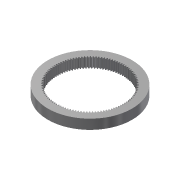
# Autodesk Inventor part: ring2
Saved by Autodesk Inventor 2018 (Build 220112000, 112)
## iProperties
Created: 2019-12-31
Part Number: ring2
Material: Steel
Document SubType Name: Modeling
Designer: louis
Categories: <?xml version="1.0" encoding="UTF-16"?> <MemberInstance><Categories><FamilyTemplate><FamilyTemplateParameter ValueType="xs:double" Id="1" ObjectReferenceKey="da_z" ObjectType="kUserParameterObject"/><FamilyTemplateParameter ValueType="xs:double" Id="2" ObjectReferenceKey="da_b" ObjectType="kUserParameterObject"/><FamilyTemplateParameter ValueType="xs:double" Id="3" ObjectReferenceKey="da_beta" ObjectType="kUserParameterObject"/><FamilyTemplateParameter ValueType="xs:double" Id="4" ObjectReferenceKey="da_da" ObjectType="kUserParameterObject"/><FamilyTemplateParameter ValueType="xs:double" Id="5" ObjectReferenceKey="da_aw" ObjectType="kUserParameterObject"/><FamilyTemplateParameter ValueType="xs:string" Id="6" ObjectReferenceKey="EAIAABAAAACIAQAAAAAAAIAAAAAAAAAA" ObjectType="83910656" SubObjectId="SurfaceGeometry"/></FamilyTemplate><ParamToTemplateMap><ParamToTemplate CategoryParameter="//CategoryParameter[@InternalName='046C89C9-8512-4d59-83FE-43B91F4F132A']" TemplateParameter="1"/><ParamToTemplate CategoryParameter="//CategoryParameter[@InternalName='2552DF32-E462-4b46-AEBF-C6C7768E72AC']" TemplateParameter="2"/><ParamToTemplate CategoryParameter="//CategoryParameter[@InternalName='C9EE641D-15FC-4fae-A226-E94C4372FDD7']" TemplateParameter="3"/><ParamToTemplate><ParamToTemplate CategoryParameter="//CategoryParameter[@InternalName='00B6519A-459B-49c7-AD84-2E56D39A5744']" ConstantValue="0.000000"/></ParamToTemplate><ParamToTemplate><ParamToTemplate CategoryParameter="//CategoryParameter[@InternalName='04B31F0E-C7A6-4894-AA32-9629BEFACF47']" ConstantValue="1.000000"/></ParamToTemplate><ParamToTemplate><ParamToTemplate CategoryParameter="//CategoryParameter[@InternalName='43CBEC2E-7847-49e7-A936-2F7889FCB2D9']" ConstantValue="0.250000"/></ParamToTemplate><ParamToTemplate><ParamToTemplate CategoryParameter="//CategoryParameter[@InternalName='B1EFC894-105D-4ebd-86BF-FA20ED196853']" ConstantValue="0.350000"/></ParamToTemplate><ParamToTemplate><ParamToTemplate CategoryParameter="//CategoryParameter[@InternalName='51175063-3D10-4879-93E8-6246FE8B403D']" ConstantValue="2060000000.000000"/></ParamToTemplate><ParamToTemplate><ParamToTemplate CategoryParameter="//CategoryParameter[@InternalName='A3A52E27-4454-46a9-B0BD-C932399B70AF']" ConstantValue="0.300000"/></ParamToTemplate><ParamToTemplate><ParamToTemplate CategoryParameter="//CategoryParameter[@InternalName='91B76062-C214-41d9-B1B9-14D2AB99603D']" ConstantValue="0.100000"/></ParamToTemplate><ParamToTemplate><ParamToTemplate CategoryParameter="//CategoryParameter[@InternalName='374E806E-8B8A-4dda-A9AA-1039D6500AD2']" ConstantValue="10.000000"/></ParamToTemplate><ParamToTemplate><ParamToTemplate CategoryParameter="//CategoryParameter[@InternalName='2D373A89-B862-43d6-8D0B-0CBF12AB9F6C']" ConstantValue="0.349066"/></ParamToTemplate><ParamToTemplate CategoryParameter="//CategoryParameter[@InternalName='37777632-D6A2-4fac-9D53-DB8ACD95C989']" TemplateParameter="4"/><ParamToTemplate CategoryParameter="//CategoryParameter[@InternalName='FD1017F1-B727-4f7e-9707-0F86F1FF9423']" TemplateParameter="5"/><ParamToTemplate><ParamToTemplate CategoryParameter="//CategoryParameter[@InternalName='9E1B4470-B2D3-4ff1-B813-535BB4CDF51A']" ConstantValue="3520000.000000"/></ParamToTemplate><ParamToTemplate><ParamToTemplate CategoryParameter="//CategoryParameter[@InternalName='F8452263-BFF6-458c-9FB1-07C4B99E95CD']" ConstantValue="11400000.000000"/></ParamToTemplate><ParamToTemplate><ParamToTemplate CategoryParameter="//CategoryParameter[@InternalName='3E3BB259-FD49-497f-8171-6EBC954A3479']" ConstantValue="2.000000"/></ParamToTemplate><ParamToTemplate CategoryParameter="//CategoryParameter[@InternalName='27C3BAF2-7550-4e4b-AE2C-0DB134B7D9B7']" TemplateParameter="6"/></ParamToTemplateMap><Category DisplayName="Gear" InternalName="DC85795E-93AB-48d5-8EEE-5A27447B64BD" Mnemonic="Gear"><CategoryParameter DisplayName="z" InternalName="046C89C9-8512-4d59-83FE-43B91F4F132A" Mnemonic="z"/><CategoryParameter DisplayName="b" InternalName="2552DF32-E462-4b46-AEBF-C6C7768E72AC" Mnemonic="b"/><CategoryParameter DisplayName="||b|" InternalName="C9EE641D-15FC-4fae-A226-E94C4372FDD7" Mnemonic="beta"/><CategoryParameter DisplayName="x" InternalName="00B6519A-459B-49c7-AD84-2E56D39A5744" Mnemonic="x"/><CategoryParameter DisplayName="a*" InternalName="04B31F0E-C7A6-4894-AA32-9629BEFACF47" Mnemonic="a"/><CategoryParameter DisplayName="c*" InternalName="43CBEC2E-7847-49e7-A936-2F7889FCB2D9" Mnemonic="c"/><CategoryParameter DisplayName="r|.f|*" InternalName="B1EFC894-105D-4ebd-86BF-FA20ED196853" Mnemonic="rf"/><CategoryParameter DisplayName="E" InternalName="51175063-3D10-4879-93E8-6246FE8B403D" Mnemonic="E"/><CategoryParameter DisplayName="||m|" InternalName="A3A52E27-4454-46a9-B0BD-C932399B70AF" Mnemonic="mi"/><Category DisplayName="SpurGear" InternalName="26C5A22E-A91E-4dfd-A3B3-23CCAFAE1764" Mnemonic="SpurGear"><CategoryParameter DisplayName="m" InternalName="91B76062-C214-41d9-B1B9-14D2AB99603D" Mnemonic="m"/><CategoryParameter DisplayName="P" InternalName="374E806E-8B8A-4dda-A9AA-1039D6500AD2" Mnemonic="PP"/><CategoryParameter DisplayName="||a|" InternalName="2D373A89-B862-43d6-8D0B-0CBF12AB9F6C" Mnemonic="alpha"/><CategoryParameter DisplayName="d|.a|" InternalName="37777632-D6A2-4fac-9D53-DB8ACD95C989" Mnemonic="da"/><CategoryParameter DisplayName="a|.w|" InternalName="FD1017F1-B727-4f7e-9707-0F86F1FF9423" Mnemonic="aw"/><CategoryParameter DisplayName="||s||.Flim|" InternalName="9E1B4470-B2D3-4ff1-B813-535BB4CDF51A" Mnemonic="sFlim"/><CategoryParameter DisplayName="||s||.Hlim|" InternalName="F8452263-BFF6-458c-9FB1-07C4B99E95CD" Mnemonic="sHlim"/><CategoryParameter DisplayName="類型" InternalName="3E3BB259-FD49-497f-8171-6EBC954A3479" Mnemonic="type"/><CategoryParameter DisplayName="PitchDiameter" InternalName="27C3BAF2-7550-4e4b-AE2C-0DB134B7D9B7" Mnemonic="IDS_PITCHDIAM"/></Category></Category></Categories></MemberInstance>
Density: 1 g/cm^3
Appearance: Steel
CustomPartVersion: 1
Author: louis
Autodesk Inventor part; units mm, degrees
sketch "Sketch1" plane through (0, 0, 0) normal (0, 0, 1) x (1, 0, 0)
  circle A0 centre (0, 0) radius 53.5
  dimension "d0" = 107
  constraints: 1 centre point
  measures "d0" diameter of A0
extrude "Extrusion1" add sketch "Sketch1" along normal blind 15
ref_plane "Work Plane2" through (0, 0, 7.5) normal (0, 0, 1) x (1, 0, 0)
sketch "Sketch2" plane through (0, 0, 0) normal (0, 0, -1) x (-1, 0, 0)
  circle A0 centre (0, 0) radius 53.5 projected
  circle A1 centre (0, 0) radius 52.5
  dimension "d3" = 105
  constraints: 1 centre point, 1 coincident
  measures "d3" diameter of A1
surface extrude "節圓直徑" sketch "Sketch2" against normal through all shown no curves A1
ref_plane "Work Plane8" through (0, 0, 0) normal (0.9995524, 0.0299155, 0) x (0, 0, 1)
ref_plane "Work Plane9" through (0, 0, 0) normal (1, 0, 0) x (0, 1, 0)
spur gear teeth "正齒輪" teeth 105 pitch diameter 105 tip diameter 107 root diameter 102.5 face width 15 start plane through (0, 0, 0) normal (0, 0, -1) x (-1, 0, 0)
sketch "草圖4" plane through (0, 0, 15) normal (0, 0, 1) x (1, 0, 0)
  arc A0 (-3.5989, 53.3788) -> (-4.2121, 51.0766) centre (9.7781, 48.5831) ccw projected
  arc A1 (-4.2121, 51.0766) -> (-4.9757, 51.0079) centre (0, 0) ccw projected
  arc A2 (-4.9757, 51.0079) -> (-5.9901, 53.1636) centre (-18.2958, 46.0564) ccw projected
  arc A3 (-5.9901, 53.1636) -> (-6.7847, 53.068) centre (0, 0) ccw projected
  arc A4 (-6.7847, 53.068) -> (-7.2591, 50.7333) centre (6.8551, 49.0809) ccw projected
  arc A5 (-7.2591, 50.7333) -> (-8.0173, 50.619) centre (0, 0) ccw projected
  arc A6 (-8.0173, 50.619) -> (-9.1588, 52.7102) centre (-21.0174, 44.8798) ccw projected
  arc A7 (-9.1588, 52.7102) -> (-9.9463, 52.5673) centre (0, 0) ccw projected
  arc A8 (-9.9463, 52.5673) -> (-10.2802, 50.2084) centre (3.9076, 49.403) ccw projected
  arc A9 (-10.2802, 50.2084) -> (-11.0301, 50.049) centre (0, 0) ccw projected
  arc A10 (-11.0301, 50.049) -> (-12.2947, 52.0681) centre (-23.6638, 43.5425) ccw projected
  arc A11 (-12.2947, 52.0681) -> (-13.0722, 51.8784) centre (0, 0) ccw projected
  arc A12 (-13.0722, 51.8784) -> (-13.2645, 49.5037) centre (0.9461, 49.5483) ccw projected
  arc A13 (-13.2645, 49.5037) -> (-14.0035, 49.2997) centre (0, 0) ccw projected
  arc A14 (-14.0035, 49.2997) -> (-15.3866, 51.2397) centre (-26.2255, 42.0494) ccw projected
  arc A15 (-15.3866, 51.2397) -> (-16.1514, 51.0038) centre (0, 0) ccw projected
  arc A16 (-16.1514, 51.0038) -> (-16.2013, 48.6218) centre (-2.0188, 49.5162) ccw projected
  arc A17 (-16.2013, 48.6218) -> (-16.9268, 48.374) centre (0, 0) ccw projected
  arc A18 (-16.9268, 48.374) -> (-18.4234, 50.2278) centre (-28.6933, 40.4057) ccw projected
  arc A19 (-18.4234, 50.2278) -> (-19.1727, 49.9466) centre (0, 0) ccw projected
  arc A20 (-19.1727, 49.9466) -> (-19.08, 47.5659) centre (-4.9764, 49.3068) ccw projected
  arc A21 (-19.08, 47.5659) -> (-19.7895, 47.2751) centre (0, 0) ccw projected
  arc A22 (-19.7895, 47.2751) -> (-21.3942, 49.0361) centre (-31.0583, 38.6174) ccw projected
  arc A23 (-21.3942, 49.0361) -> (-22.1254, 48.7105) centre (0, 0) ccw projected
  arc A24 (-22.1254, 48.7105) -> (-21.8905, 46.3397) centre (-7.9163, 48.921) ccw projected
  arc A25 (-21.8905, 46.3397) -> (-22.5813, 46.007) centre (0, 0) ccw projected
  arc A26 (-22.5813, 46.007) -> (-24.2885, 47.6688) centre (-33.3122, 36.6909) ccw projected
  arc A27 (-24.2885, 47.6688) -> (-24.9989, 47.3002) centre (0, 0) ccw projected
  arc A28 (-24.9989, 47.3002) -> (-24.6227, 44.9476) centre (-10.8278, 48.36) ccw projected
  arc A29 (-24.6227, 44.9476) -> (-25.2923, 44.5742) centre (0, 0) ccw projected
  arc A30 (-25.2923, 44.5742) -> (-27.0958, 46.131) centre (-35.4469, 34.633) ccw projected
  arc A31 (-27.0958, 46.131) -> (-27.7829, 45.7205) centre (0, 0) ccw projected
  arc A32 (-27.7829, 45.7205) -> (-27.2666, 43.3946) centre (-13.7005, 47.6259) ccw projected
  arc A33 (-27.2666, 43.3946) -> (-27.9128, 42.9819) centre (0, 0) ccw projected
  arc A34 (-27.9128, 42.9819) -> (-29.8061, 44.428) centre (-37.4546, 32.4512) ccw projected
  arc A35 (-29.8061, 44.428) -> (-30.4674, 43.9771) centre (0, 0) ccw projected
  arc A36 (-30.4674, 43.9771) -> (-29.813, 41.6863) centre (-16.5242, 46.7213) ccw projected
  arc A37 (-29.813, 41.6863) -> (-30.4333, 41.2356) centre (0, 0) ccw projected
  arc A38 (-30.4333, 41.2356) -> (-32.4098, 42.5659) centre (-39.3283, 30.1531) ccw projected
  arc A39 (-32.4098, 42.5659) -> (-33.0429, 42.0763) centre (0, 0) ccw projected
  arc A40 (-33.0429, 42.0763) -> (-32.2527, 39.8287) centre (-19.2888, 45.6494) ccw projected
  arc A41 (-32.2527, 39.8287) -> (-32.8449, 39.3418) centre (0, 0) ccw projected
  arc A42 (-32.8449, 39.3418) -> (-34.8974, 40.5515) centre (-41.0612, 27.7472) ccw projected
  arc A43 (-34.8974, 40.5515) -> (-35.5001, 40.0249) centre (0, 0) ccw projected
  arc A44 (-35.5001, 40.0249) -> (-34.5769, 37.8286) centre (-21.9843, 44.4142) ccw projected
  arc A45 (-34.5769, 37.8286) -> (-35.1389, 37.3071) centre (0, 0) ccw projected
  arc A46 (-35.1389, 37.3071) -> (-37.2601, 38.3919) centre (-42.6471, 25.2419) ccw projected
  arc A47 (-37.2601, 38.3919) -> (-37.8302, 37.8302) centre (0, 0) ccw projected
  arc A48 (-37.8302, 37.8302) -> (-36.7773, 35.6931) centre (-24.6011, 43.0199) ccw projected
  arc A49 (-36.7773, 35.6931) -> (-37.3071, 35.1389) centre (0, 0) ccw projected
  arc A50 (-37.3071, 35.1389) -> (-39.4894, 36.0949) centre (-44.0803, 22.6462) ccw projected
  arc A51 (-39.4894, 36.0949) -> (-40.0249, 35.5001) centre (0, 0) ccw projected
  arc A52 (-40.0249, 35.5001) -> (-38.8461, 33.4297) centre (-27.1298, 41.4717) ccw projected
  arc A53 (-38.8461, 33.4297) -> (-39.3418, 32.8449) centre (0, 0) ccw projected
  arc A54 (-39.3418, 32.8449) -> (-41.5773, 33.6686) centre (-45.3558, 19.9695) ccw projected
  arc A55 (-41.5773, 33.6686) -> (-42.0763, 33.0429) centre (0, 0) ccw projected
  arc A56 (-42.0763, 33.0429) -> (-40.7758, 31.0467) centre (-29.5614, 39.775) ccw projected
  arc A57 (-40.7758, 31.0467) -> (-41.2356, 30.4333) centre (0, 0) ccw projected
  arc A58 (-41.2356, 30.4333) -> (-43.5164, 31.1219) centre (-46.4689, 17.2213) ccw projected
  arc A59 (-43.5164, 31.1219) -> (-43.9771, 30.4674) centre (0, 0) ccw projected
  arc A60 (-43.9771, 30.4674) -> (-42.5595, 28.5526) centre (-31.8872, 37.9359) ccw projected
  arc A61 (-42.5595, 28.5526) -> (-42.9819, 27.9128) centre (0, 0) ccw projected
  arc A62 (-42.9819, 27.9128) -> (-45.2997, 28.4637) centre (-47.4156, 14.4114) ccw projected
  arc A63 (-45.2997, 28.4637) -> (-45.7205, 27.7829) centre (0, 0) ccw projected
  arc A64 (-45.7205, 27.7829) -> (-44.1909, 25.9563) centre (-34.0989, 35.961) ccw projected
  arc A65 (-44.1909, 25.9563) -> (-44.5742, 25.2923) centre (0, 0) ccw projected
  arc A66 (-44.5742, 25.2923) -> (-46.9209, 25.7037) centre (-48.1926, 11.55) ccw projected
  arc A67 (-46.9209, 25.7037) -> (-47.3002, 24.9989) centre (0, 0) ccw projected
  arc A68 (-47.3002, 24.9989) -> (-45.6641, 23.267) centre (-36.1885, 33.8574) ccw projected
  arc A69 (-45.6641, 23.267) -> (-46.007, 22.5813) centre (0, 0) ccw projected
  arc A70 (-46.007, 22.5813) -> (-48.3741, 22.8516) centre (-48.7971, 8.6472) ccw projected
  arc A71 (-48.3741, 22.8516) -> (-48.7105, 22.1254) centre (0, 0) ccw projected
  arc A72 (-48.7105, 22.1254) -> (-46.9738, 20.4945) centre (-38.1485, 31.6326) ccw projected
  arc A73 (-46.9738, 20.4945) -> (-47.2751, 19.7895) centre (0, 0) ccw projected
  arc A74 (-47.2751, 19.7895) -> (-49.6542, 19.9177) centre (-49.2269, 5.7135) ccw projected
  arc A75 (-49.6542, 19.9177) -> (-49.9466, 19.1727) centre (0, 0) ccw projected
  arc A76 (-49.9466, 19.1727) -> (-48.1154, 17.6486) centre (-39.972, 29.2945) ccw projected
  arc A77 (-48.1154, 17.6486) -> (-48.374, 16.9268) centre (0, 0) ccw projected
  arc A78 (-48.374, 16.9268) -> (-50.7564, 16.9125) centre (-49.4804, 2.7593) ccw projected
  arc A79 (-50.7564, 16.9125) -> (-51.0038, 16.1514) centre (0, 0) ccw projected
  arc A80 (-51.0038, 16.1514) -> (-49.0847, 14.7395) centre (-41.6524, 26.8516) ccw projected
  arc A81 (-49.0847, 14.7395) -> (-49.2997, 14.0035) centre (0, 0) ccw projected
  arc A82 (-49.2997, 14.0035) -> (-51.677, 13.8468) centre (-49.5569, -0.2048) ccw projected
  arc A83 (-51.677, 13.8468) -> (-51.8784, 13.0722) centre (0, 0) ccw projected
  arc A84 (-51.8784, 13.0722) -> (-49.8784, 11.7776) centre (-43.1837, 24.3125) ccw projected
  arc A85 (-49.8784, 11.7776) -> (-50.049, 11.0301) centre (0, 0) ccw projected
  arc A86 (-50.049, 11.0301) -> (-52.4126, 10.7315) centre (-49.4559, -3.1681) ccw projected
  arc A87 (-52.4126, 10.7315) -> (-52.5673, 9.9463) centre (0, 0) ccw projected
  arc A88 (-52.5673, 9.9463) -> (-50.4934, 8.7736) centre (-44.5604, 21.6865) ccw projected
  arc A89 (-50.4934, 8.7736) -> (-50.619, 8.0173) centre (0, 0) ccw projected
  arc A90 (-50.619, 8.0173) -> (-52.9606, 7.5778) centre (-49.178, -6.1201) ccw projected
  arc A91 (-52.9606, 7.5778) -> (-53.068, 6.7847) centre (0, 0) ccw projected
  arc A92 (-53.068, 6.7847) -> (-50.9278, 5.7382) centre (-45.7775, 18.9827) ccw projected
  arc A93 (-50.9278, 5.7382) -> (-51.0079, 4.9757) centre (0, 0) ccw projected
  arc A94 (-51.0079, 4.9757) -> (-53.319, 4.397) centre (-48.7239, -9.0502) ccw projected
  arc A95 (-53.319, 4.397) -> (-53.3788, 3.5989) centre (0, 0) ccw projected
  arc A96 (-53.3788, 3.5989) -> (-51.1798, 2.6822) centre (-46.8308, 16.2111) ccw projected
  arc A97 (-51.1798, 2.6822) -> (-51.2142, 1.9163) centre (0, 0) ccw projected
  arc A98 (-51.2142, 1.9163) -> (-53.4865, 1.2004) centre (-48.0955, -11.9479) ccw projected
  arc A99 (-53.4865, 1.2004) -> (-53.4985, 0.4002) centre (0, 0) ccw projected
  arc A100 (-53.4985, 0.4002) -> (-51.2486, -0.3833) centre (-47.7165, 13.3814) ccw projected
  arc A101 (-51.2486, -0.3833) -> (-51.2371, -1.15) centre (0, 0) ccw projected
  arc A102 (-51.2371, -1.15) -> (-53.4626, -2.0004) centre (-47.2948, -14.8029) ccw projected
  arc A103 (-53.4626, -2.0004) -> (-53.4267, -2.8) centre (0, 0) ccw projected
  arc A104 (-53.4267, -2.8) -> (-51.1339, -3.4475) centre (-48.4314, 10.5038) ccw projected
  arc A105 (-51.1339, -3.4475) -> (-51.0766, -4.2121) centre (0, 0) ccw projected
  arc A106 (-51.0766, -4.2121) -> (-53.2473, -5.1941) centre (-46.3249, -17.6048) ccw projected
  arc A107 (-53.2473, -5.1941) -> (-53.1636, -5.9901) centre (0, 0) ccw projected
  arc A108 (-53.1636, -5.9901) -> (-50.8362, -6.4994) centre (-48.9729, 7.5886) ccw projected
  arc A109 (-50.8362, -6.4994) -> (-50.7333, -7.2591) centre (0, 0) ccw projected
  arc A110 (-50.7333, -7.2591) -> (-52.8413, -8.3692) centre (-45.1892, -20.3437) ccw projected
  arc A111 (-52.8413, -8.3692) -> (-52.7102, -9.1588) centre (0, 0) ccw projected
  arc A112 (-52.7102, -9.1588) -> (-50.3565, -9.528) centre (-49.339, 4.6462) ccw projected
  arc A113 (-50.3565, -9.528) -> (-50.2084, -10.2802) centre (0, 0) ccw projected
  arc A114 (-50.2084, -10.2802) -> (-52.2462, -11.5144) centre (-43.8916, -23.0098) ccw projected
  arc A115 (-52.2462, -11.5144) -> (-52.0681, -12.2947) centre (0, 0) ccw projected
  arc A116 (-52.0681, -12.2947) -> (-49.6966, -12.5224) centre (-49.5286, 1.6872) ccw projected
  arc A117 (-49.6966, -12.5224) -> (-49.5037, -13.2645) centre (0, 0) ccw projected
  arc A118 (-49.5037, -13.2645) -> (-51.4641, -14.6183) centre (-42.437, -25.5935) ccw projected
  arc A119 (-51.4641, -14.6183) -> (-51.2397, -15.3866) centre (0, 0) ccw projected
  arc A120 (-51.2397, -15.3866) -> (-48.8587, -15.4721) centre (-49.5408, -1.2778) ccw projected
  arc A121 (-48.8587, -15.4721) -> (-48.6218, -16.2013) centre (0, 0) ccw projected
  arc A122 (-48.6218, -16.2013) -> (-50.4978, -17.6699) centre (-40.8305, -28.0856) ccw projected
  arc A123 (-50.4978, -17.6699) -> (-50.2278, -18.4234) centre (0, 0) ccw projected
  arc A124 (-50.2278, -18.4234) -> (-47.846, -18.3664) centre (-49.3757, -4.2383) ccw projected
  arc A125 (-47.846, -18.3664) -> (-47.5659, -19.08) centre (0, 0) ccw projected
  arc A126 (-47.5659, -19.08) -> (-49.3506, -20.6583) centre (-39.0777, -30.4772) ccw projected
  arc A127 (-49.3506, -20.6583) -> (-49.0361, -21.3942) centre (0, 0) ccw projected
  arc A128 (-49.0361, -21.3942) -> (-46.662, -21.1949) centre (-49.0339, -7.1836) ccw projected
  arc A129 (-46.662, -21.1949) -> (-46.3397, -21.8905) centre (0, 0) ccw projected
  arc A130 (-46.3397, -21.8905) -> (-48.0269, -23.5727) centre (-37.1851, -32.7596) ccw projected
  arc A131 (-48.0269, -23.5727) -> (-47.6688, -24.2885) centre (0, 0) ccw projected
  arc A132 (-47.6688, -24.2885) -> (-45.3109, -23.9475) centre (-48.5165, -10.1031) ccw projected
  arc A133 (-45.3109, -23.9475) -> (-44.9476, -24.6227) centre (0, 0) ccw projected
  arc A134 (-44.9476, -24.6227) -> (-46.5312, -26.4027) centre (-35.1594, -34.9248) ccw projected
  arc A135 (-46.5312, -26.4027) -> (-46.131, -27.0958) centre (0, 0) ccw projected
  arc A136 (-46.131, -27.0958) -> (-43.7977, -26.6144) centre (-47.8255, -12.9865) ccw projected
  arc A137 (-43.7977, -26.6144) -> (-43.3946, -27.2666) centre (0, 0) ccw projected
  arc A138 (-43.3946, -27.2666) -> (-44.8689, -29.1382) centre (-33.0078, -36.965) ccw projected
  arc A139 (-44.8689, -29.1382) -> (-44.428, -29.8061) centre (0, 0) ccw projected
  arc A140 (-44.428, -29.8061) -> (-42.1276, -29.1861) centre (-46.9632, -15.8235) ccw projected
  arc A141 (-42.1276, -29.1861) -> (-41.6863, -29.813) centre (0, 0) ccw projected
  arc A142 (-41.6863, -29.813) -> (-43.046, -31.7694) centre (-30.7381, -38.8728) ccw projected
  arc A143 (-43.046, -31.7694) -> (-42.5659, -32.4098) centre (0, 0) ccw projected
  arc A144 (-42.5659, -32.4098) -> (-40.3068, -31.6532) centre (-45.9329, -18.6037) ccw projected
  arc A145 (-40.3068, -31.6532) -> (-39.8287, -32.2527) centre (0, 0) ccw projected
  arc A146 (-39.8287, -32.2527) -> (-41.069, -34.2868) centre (-28.3583, -40.6415) ccw projected
  arc A147 (-41.069, -34.2868) -> (-40.5515, -34.8974) centre (0, 0) ccw projected
  arc A148 (-40.5515, -34.8974) -> (-38.3416, -34.0071) centre (-44.7381, -21.3174) ccw projected
  arc A149 (-38.3416, -34.0071) -> (-37.8286, -34.5769) centre (0, 0) ccw projected
  arc A150 (-37.8286, -34.5769) -> (-38.945, -36.6816) centre (-25.877, -42.2647) ccw projected
  arc A151 (-38.945, -36.6816) -> (-38.3919, -37.2601) centre (0, 0) ccw projected
  arc A152 (-38.3919, -37.2601) -> (-36.2392, -36.2392) centre (-43.3831, -23.9548) ccw projected
  arc A153 (-36.2392, -36.2392) -> (-35.6931, -36.7773) centre (0, 0) ccw projected
  arc A154 (-35.6931, -36.7773) -> (-36.6816, -38.945) centre (-23.3031, -43.7366) ccw projected
  arc A155 (-36.6816, -38.945) -> (-36.0949, -39.4894) centre (0, 0) ccw projected
  arc A156 (-36.0949, -39.4894) -> (-34.0071, -38.3416) centre (-41.8729, -26.5064) ccw projected
  arc A157 (-34.0071, -38.3416) -> (-33.4297, -38.8461) centre (0, 0) ccw projected
  arc A158 (-33.4297, -38.8461) -> (-34.2868, -41.069) centre (-20.6458, -45.052) ccw projected
  arc A159 (-34.2868, -41.069) -> (-33.6686, -41.5773) centre (0, 0) ccw projected
  arc A160 (-33.6686, -41.5773) -> (-31.6532, -40.3068) centre (-40.2127, -28.9631) ccw projected
  arc A161 (-31.6532, -40.3068) -> (-31.0467, -40.7758) centre (0, 0) ccw projected
  arc A162 (-31.0467, -40.7758) -> (-31.7694, -43.046) centre (-17.9145, -46.206) ccw projected
  arc A163 (-31.7694, -43.046) -> (-31.1219, -43.5164) centre (0, 0) ccw projected
  arc A164 (-31.1219, -43.5164) -> (-29.1861, -42.1276) centre (-38.4087, -31.3162) ccw projected
  arc A165 (-29.1861, -42.1276) -> (-28.5526, -42.5595) centre (0, 0) ccw projected
  arc A166 (-28.5526, -42.5595) -> (-29.1382, -44.8689) centre (-15.1191, -47.1947) ccw projected
  arc A167 (-29.1382, -44.8689) -> (-28.4637, -45.2997) centre (0, 0) ccw projected
  arc A168 (-28.4637, -45.2997) -> (-26.6144, -43.7977) centre (-36.4671, -33.5571) ccw projected
  arc A169 (-26.6144, -43.7977) -> (-25.9563, -44.1909) centre (0, 0) ccw projected
  arc A170 (-25.9563, -44.1909) -> (-26.4027, -46.5312) centre (-12.2696, -48.0144) ccw projected
  arc A171 (-26.4027, -46.5312) -> (-25.7037, -46.9209) centre (0, 0) ccw projected
  arc A172 (-25.7037, -46.9209) -> (-23.9475, -45.3109) centre (-34.3949, -35.6779) ccw projected
  arc A173 (-23.9475, -45.3109) -> (-23.267, -45.6641) centre (0, 0) ccw projected
  arc A174 (-23.267, -45.6641) -> (-23.5727, -48.0269) centre (-9.3762, -48.6622) ccw projected
  arc A175 (-23.5727, -48.0269) -> (-22.8516, -48.3741) centre (0, 0) ccw projected
  arc A176 (-22.8516, -48.3741) -> (-21.1949, -46.662) centre (-32.1997, -37.671) ccw projected
  arc A177 (-21.1949, -46.662) -> (-20.4945, -46.9738) centre (0, 0) ccw projected
  arc A178 (-20.4945, -46.9738) -> (-20.6583, -49.3506) centre (-6.4492, -49.1359) ccw projected
  arc A179 (-20.6583, -49.3506) -> (-19.9177, -49.6542) centre (0, 0) ccw projected
  arc A180 (-19.9177, -49.6542) -> (-18.3664, -47.846) centre (-29.8892, -39.5293) ccw projected
  arc A181 (-18.3664, -47.846) -> (-17.6486, -48.1154) centre (0, 0) ccw projected
  arc A182 (-17.6486, -48.1154) -> (-17.6699, -50.4978) centre (-3.4992, -49.4336) ccw projected
  arc A183 (-17.6699, -50.4978) -> (-16.9125, -50.7564) centre (0, 0) ccw projected
  arc A184 (-16.9125, -50.7564) -> (-15.4721, -48.8587) centre (-27.4717, -41.246) ccw projected
  arc A185 (-15.4721, -48.8587) -> (-14.7395, -49.0847) centre (0, 0) ccw projected
  arc A186 (-14.7395, -49.0847) -> (-14.6183, -51.4641) centre (-0.5366, -49.5544) ccw projected
  arc A187 (-14.6183, -51.4641) -> (-13.8468, -51.677) centre (0, 0) ccw projected
  arc A188 (-13.8468, -51.677) -> (-12.5224, -49.6966) centre (-24.9558, -42.8151) ccw projected
  arc A189 (-12.5224, -49.6966) -> (-11.7776, -49.8784) centre (0, 0) ccw projected
  arc A190 (-11.7776, -49.8784) -> (-11.5144, -52.2462) centre (2.428, -49.4978) ccw projected
  arc A191 (-11.5144, -52.2462) -> (-10.7315, -52.4126) centre (0, 0) ccw projected
  arc A192 (-10.7315, -52.4126) -> (-9.528, -50.3565) centre (-22.3506, -44.2309) ccw projected
  arc A193 (-9.528, -50.3565) -> (-8.7736, -50.4934) centre (0, 0) ccw projected
  arc A194 (-8.7736, -50.4934) -> (-8.3692, -52.8413) centre (5.3838, -49.264) ccw projected
  arc A195 (-8.3692, -52.8413) -> (-7.5778, -52.9606) centre (0, 0) ccw projected
  arc A196 (-7.5778, -52.9606) -> (-6.4994, -50.8362) centre (-19.6654, -45.4884) ccw projected
  arc A197 (-6.4994, -50.8362) -> (-5.7382, -50.9278) centre (0, 0) ccw projected
  arc A198 (-5.7382, -50.9278) -> (-5.1941, -53.2473) centre (8.3203, -48.8539) ccw projected
  arc A199 (-5.1941, -53.2473) -> (-4.397, -53.319) centre (0, 0) ccw projected
  arc A200 (-4.397, -53.319) -> (-3.4475, -51.1339) centre (-16.9098, -46.5831) ccw projected
  arc A201 (-3.4475, -51.1339) -> (-2.6822, -51.1798) centre (0, 0) ccw projected
  arc A202 (-2.6822, -51.1798) -> (-2.0004, -53.4626) centre (11.2271, -48.2688) ccw projected
  arc A203 (-2.0004, -53.4626) -> (-1.2004, -53.4865) centre (0, 0) ccw projected
  arc A204 (-1.2004, -53.4865) -> (-0.3833, -51.2486) centre (-14.0937, -47.511) ccw projected
  arc A205 (-0.3833, -51.2486) -> (0.3833, -51.2486) centre (0, 0) ccw projected
  arc A206 (0.3833, -51.2486) -> (1.2004, -53.4865) centre (14.0937, -47.511) ccw projected
  arc A207 (1.2004, -53.4865) -> (2.0004, -53.4626) centre (0, 0) ccw projected
  arc A208 (2.0004, -53.4626) -> (2.6822, -51.1798) centre (-11.2271, -48.2688) ccw projected
  arc A209 (2.6822, -51.1798) -> (3.4475, -51.1339) centre (0, 0) ccw projected
  arc A210 (3.4475, -51.1339) -> (4.397, -53.319) centre (16.9098, -46.5831) ccw projected
  arc A211 (4.397, -53.319) -> (5.1941, -53.2473) centre (0, 0) ccw projected
  arc A212 (5.1941, -53.2473) -> (5.7382, -50.9278) centre (-8.3203, -48.8539) ccw projected
  arc A213 (5.7382, -50.9278) -> (6.4994, -50.8362) centre (0, 0) ccw projected
  arc A214 (6.4994, -50.8362) -> (7.5778, -52.9606) centre (19.6654, -45.4884) ccw projected
  arc A215 (7.5778, -52.9606) -> (8.3692, -52.8413) centre (0, 0) ccw projected
  arc A216 (8.3692, -52.8413) -> (8.7736, -50.4934) centre (-5.3838, -49.264) ccw projected
  arc A217 (8.7736, -50.4934) -> (9.528, -50.3565) centre (0, 0) ccw projected
  arc A218 (9.528, -50.3565) -> (10.7315, -52.4126) centre (22.3506, -44.2309) ccw projected
  arc A219 (10.7315, -52.4126) -> (11.5144, -52.2462) centre (0, 0) ccw projected
  arc A220 (11.5144, -52.2462) -> (11.7776, -49.8784) centre (-2.428, -49.4978) ccw projected
  arc A221 (11.7776, -49.8784) -> (12.5224, -49.6966) centre (0, 0) ccw projected
  arc A222 (12.5224, -49.6966) -> (13.8468, -51.677) centre (24.9558, -42.8151) ccw projected
  arc A223 (13.8468, -51.677) -> (14.6183, -51.4641) centre (0, 0) ccw projected
  arc A224 (14.6183, -51.4641) -> (14.7395, -49.0847) centre (0.5366, -49.5544) ccw projected
  arc A225 (14.7395, -49.0847) -> (15.4721, -48.8587) centre (0, 0) ccw projected
  arc A226 (15.4721, -48.8587) -> (16.9125, -50.7564) centre (27.4717, -41.246) ccw projected
  arc A227 (16.9125, -50.7564) -> (17.6699, -50.4978) centre (0, 0) ccw projected
  arc A228 (17.6699, -50.4978) -> (17.6486, -48.1154) centre (3.4992, -49.4336) ccw projected
  arc A229 (17.6486, -48.1154) -> (18.3664, -47.846) centre (0, 0) ccw projected
  arc A230 (18.3664, -47.846) -> (19.9177, -49.6542) centre (29.8892, -39.5293) ccw projected
  arc A231 (19.9177, -49.6542) -> (20.6583, -49.3506) centre (0, 0) ccw projected
  arc A232 (20.6583, -49.3506) -> (20.4945, -46.9738) centre (6.4492, -49.1359) ccw projected
  arc A233 (20.4945, -46.9738) -> (21.1949, -46.662) centre (0, 0) ccw projected
  arc A234 (21.1949, -46.662) -> (22.8516, -48.3741) centre (32.1997, -37.671) ccw projected
  arc A235 (22.8516, -48.3741) -> (23.5727, -48.0269) centre (0, 0) ccw projected
  arc A236 (23.5727, -48.0269) -> (23.267, -45.6641) centre (9.3762, -48.6622) ccw projected
  arc A237 (23.267, -45.6641) -> (23.9475, -45.3109) centre (0, 0) ccw projected
  arc A238 (23.9475, -45.3109) -> (25.7037, -46.9209) centre (34.3949, -35.6779) ccw projected
  arc A239 (25.7037, -46.9209) -> (26.4027, -46.5312) centre (0, 0) ccw projected
  arc A240 (26.4027, -46.5312) -> (25.9563, -44.1909) centre (12.2696, -48.0144) ccw projected
  arc A241 (25.9563, -44.1909) -> (26.6144, -43.7977) centre (0, 0) ccw projected
  arc A242 (26.6144, -43.7977) -> (28.4637, -45.2997) centre (36.4671, -33.5571) ccw projected
  arc A243 (28.4637, -45.2997) -> (29.1382, -44.8689) centre (0, 0) ccw projected
  arc A244 (29.1382, -44.8689) -> (28.5526, -42.5595) centre (15.1191, -47.1947) ccw projected
  arc A245 (28.5526, -42.5595) -> (29.1861, -42.1276) centre (0, 0) ccw projected
  arc A246 (29.1861, -42.1276) -> (31.1219, -43.5164) centre (38.4087, -31.3162) ccw projected
  arc A247 (31.1219, -43.5164) -> (31.7694, -43.046) centre (0, 0) ccw projected
  arc A248 (31.7694, -43.046) -> (31.0467, -40.7758) centre (17.9145, -46.206) ccw projected
  arc A249 (31.0467, -40.7758) -> (31.6532, -40.3068) centre (0, 0) ccw projected
  arc A250 (31.6532, -40.3068) -> (33.6686, -41.5773) centre (40.2127, -28.9631) ccw projected
  arc A251 (33.6686, -41.5773) -> (34.2868, -41.069) centre (0, 0) ccw projected
  arc A252 (34.2868, -41.069) -> (33.4297, -38.8461) centre (20.6458, -45.052) ccw projected
  arc A253 (33.4297, -38.8461) -> (34.0071, -38.3416) centre (0, 0) ccw projected
  arc A254 (34.0071, -38.3416) -> (36.0949, -39.4894) centre (41.8729, -26.5064) ccw projected
  arc A255 (36.0949, -39.4894) -> (36.6816, -38.945) centre (0, 0) ccw projected
  arc A256 (36.6816, -38.945) -> (35.6931, -36.7773) centre (23.3031, -43.7366) ccw projected
  arc A257 (35.6931, -36.7773) -> (36.2392, -36.2392) centre (0, 0) ccw projected
  arc A258 (36.2392, -36.2392) -> (38.3919, -37.2601) centre (43.3831, -23.9548) ccw projected
  arc A259 (38.3919, -37.2601) -> (38.945, -36.6816) centre (0, 0) ccw projected
  arc A260 (38.945, -36.6816) -> (37.8286, -34.5769) centre (25.877, -42.2647) ccw projected
  arc A261 (37.8286, -34.5769) -> (38.3416, -34.0071) centre (0, 0) ccw projected
  arc A262 (38.3416, -34.0071) -> (40.5515, -34.8974) centre (44.7381, -21.3174) ccw projected
  arc A263 (40.5515, -34.8974) -> (41.069, -34.2868) centre (0, 0) ccw projected
  arc A264 (41.069, -34.2868) -> (39.8287, -32.2527) centre (28.3583, -40.6415) ccw projected
  arc A265 (39.8287, -32.2527) -> (40.3068, -31.6532) centre (0, 0) ccw projected
  arc A266 (40.3068, -31.6532) -> (42.5659, -32.4098) centre (45.9329, -18.6037) ccw projected
  arc A267 (42.5659, -32.4098) -> (43.046, -31.7694) centre (0, 0) ccw projected
  arc A268 (43.046, -31.7694) -> (41.6863, -29.813) centre (30.7381, -38.8728) ccw projected
  arc A269 (41.6863, -29.813) -> (42.1276, -29.1861) centre (0, 0) ccw projected
  arc A270 (42.1276, -29.1861) -> (44.428, -29.8061) centre (46.9632, -15.8235) ccw projected
  arc A271 (44.428, -29.8061) -> (44.8689, -29.1382) centre (0, 0) ccw projected
  arc A272 (44.8689, -29.1382) -> (43.3946, -27.2666) centre (33.0078, -36.965) ccw projected
  arc A273 (43.3946, -27.2666) -> (43.7977, -26.6144) centre (0, 0) ccw projected
  arc A274 (43.7977, -26.6144) -> (46.131, -27.0958) centre (47.8255, -12.9865) ccw projected
  arc A275 (46.131, -27.0958) -> (46.5312, -26.4027) centre (0, 0) ccw projected
  arc A276 (46.5312, -26.4027) -> (44.9476, -24.6227) centre (35.1594, -34.9248) ccw projected
  arc A277 (44.9476, -24.6227) -> (45.3109, -23.9475) centre (0, 0) ccw projected
  arc A278 (45.3109, -23.9475) -> (47.6688, -24.2885) centre (48.5165, -10.1031) ccw projected
  arc A279 (47.6688, -24.2885) -> (48.0269, -23.5727) centre (0, 0) ccw projected
  arc A280 (48.0269, -23.5727) -> (46.3397, -21.8905) centre (37.1851, -32.7596) ccw projected
  arc A281 (46.3397, -21.8905) -> (46.662, -21.1949) centre (0, 0) ccw projected
  arc A282 (46.662, -21.1949) -> (49.0361, -21.3942) centre (49.0339, -7.1836) ccw projected
  arc A283 (49.0361, -21.3942) -> (49.3506, -20.6583) centre (0, 0) ccw projected
  arc A284 (49.3506, -20.6583) -> (47.5659, -19.08) centre (39.0777, -30.4772) ccw projected
  arc A285 (47.5659, -19.08) -> (47.846, -18.3664) centre (0, 0) ccw projected
  arc A286 (47.846, -18.3664) -> (50.2278, -18.4234) centre (49.3757, -4.2383) ccw projected
  arc A287 (50.2278, -18.4234) -> (50.4978, -17.6699) centre (0, 0) ccw projected
  arc A288 (50.4978, -17.6699) -> (48.6218, -16.2013) centre (40.8305, -28.0856) ccw projected
  arc A289 (48.6218, -16.2013) -> (48.8587, -15.4721) centre (0, 0) ccw projected
  arc A290 (48.8587, -15.4721) -> (51.2397, -15.3866) centre (49.5408, -1.2778) ccw projected
  arc A291 (51.2397, -15.3866) -> (51.4641, -14.6183) centre (0, 0) ccw projected
  arc A292 (51.4641, -14.6183) -> (49.5037, -13.2645) centre (42.437, -25.5935) ccw projected
  arc A293 (49.5037, -13.2645) -> (49.6966, -12.5224) centre (0, 0) ccw projected
  arc A294 (49.6966, -12.5224) -> (52.0681, -12.2947) centre (49.5286, 1.6872) ccw projected
  arc A295 (52.0681, -12.2947) -> (52.2462, -11.5144) centre (0, 0) ccw projected
  arc A296 (52.2462, -11.5144) -> (50.2084, -10.2802) centre (43.8916, -23.0098) ccw projected
  arc A297 (50.2084, -10.2802) -> (50.3565, -9.528) centre (0, 0) ccw projected
  arc A298 (50.3565, -9.528) -> (52.7102, -9.1588) centre (49.339, 4.6462) ccw projected
  arc A299 (52.7102, -9.1588) -> (52.8413, -8.3692) centre (0, 0) ccw projected
  arc A300 (52.8413, -8.3692) -> (50.7333, -7.2591) centre (45.1892, -20.3437) ccw projected
  arc A301 (50.7333, -7.2591) -> (50.8362, -6.4994) centre (0, 0) ccw projected
  arc A302 (50.8362, -6.4994) -> (53.1636, -5.9901) centre (48.9729, 7.5886) ccw projected
  arc A303 (53.1636, -5.9901) -> (53.2473, -5.1941) centre (0, 0) ccw projected
  arc A304 (53.2473, -5.1941) -> (51.0766, -4.2121) centre (46.3249, -17.6048) ccw projected
  arc A305 (51.0766, -4.2121) -> (51.1339, -3.4475) centre (0, 0) ccw projected
  arc A306 (51.1339, -3.4475) -> (53.4267, -2.8) centre (48.4314, 10.5038) ccw projected
  arc A307 (53.4267, -2.8) -> (53.4626, -2.0004) centre (0, 0) ccw projected
  arc A308 (53.4626, -2.0004) -> (51.2371, -1.15) centre (47.2948, -14.8029) ccw projected
  arc A309 (51.2371, -1.15) -> (51.2486, -0.3833) centre (0, 0) ccw projected
  arc A310 (51.2486, -0.3833) -> (53.4985, 0.4002) centre (47.7165, 13.3814) ccw projected
  arc A311 (53.4985, 0.4002) -> (53.4865, 1.2004) centre (0, 0) ccw projected
  arc A312 (53.4865, 1.2004) -> (51.2142, 1.9163) centre (48.0955, -11.9479) ccw projected
  arc A313 (51.2142, 1.9163) -> (51.1798, 2.6822) centre (0, 0) ccw projected
  arc A314 (51.1798, 2.6822) -> (53.3788, 3.5989) centre (46.8308, 16.2111) ccw projected
  arc A315 (53.3788, 3.5989) -> (53.319, 4.397) centre (0, 0) ccw projected
  arc A316 (53.319, 4.397) -> (51.0079, 4.9757) centre (48.7239, -9.0502) ccw projected
  arc A317 (51.0079, 4.9757) -> (50.9278, 5.7382) centre (0, 0) ccw projected
  arc A318 (50.9278, 5.7382) -> (53.068, 6.7847) centre (45.7775, 18.9827) ccw projected
  arc A319 (53.068, 6.7847) -> (52.9606, 7.5778) centre (0, 0) ccw projected
  arc A320 (52.9606, 7.5778) -> (50.619, 8.0173) centre (49.178, -6.1201) ccw projected
  arc A321 (50.619, 8.0173) -> (50.4934, 8.7736) centre (0, 0) ccw projected
  arc A322 (50.4934, 8.7736) -> (52.5673, 9.9463) centre (44.5604, 21.6865) ccw projected
  arc A323 (52.5673, 9.9463) -> (52.4126, 10.7315) centre (0, 0) ccw projected
  arc A324 (52.4126, 10.7315) -> (50.049, 11.0301) centre (49.4559, -3.1681) ccw projected
  arc A325 (50.049, 11.0301) -> (49.8784, 11.7776) centre (0, 0) ccw projected
  arc A326 (49.8784, 11.7776) -> (51.8784, 13.0722) centre (43.1837, 24.3125) ccw projected
  arc A327 (51.8784, 13.0722) -> (51.677, 13.8468) centre (0, 0) ccw projected
  arc A328 (51.677, 13.8468) -> (49.2997, 14.0035) centre (49.5569, -0.2048) ccw projected
  arc A329 (49.2997, 14.0035) -> (49.0847, 14.7395) centre (0, 0) ccw projected
  arc A330 (49.0847, 14.7395) -> (51.0038, 16.1514) centre (41.6524, 26.8516) ccw projected
  arc A331 (51.0038, 16.1514) -> (50.7564, 16.9125) centre (0, 0) ccw projected
  arc A332 (50.7564, 16.9125) -> (48.374, 16.9268) centre (49.4804, 2.7593) ccw projected
  arc A333 (48.374, 16.9268) -> (48.1154, 17.6486) centre (0, 0) ccw projected
  arc A334 (48.1154, 17.6486) -> (49.9466, 19.1727) centre (39.972, 29.2945) ccw projected
  arc A335 (49.9466, 19.1727) -> (49.6542, 19.9177) centre (0, 0) ccw projected
  arc A336 (49.6542, 19.9177) -> (47.2751, 19.7895) centre (49.2269, 5.7135) ccw projected
  arc A337 (47.2751, 19.7895) -> (46.9738, 20.4945) centre (0, 0) ccw projected
  arc A338 (46.9738, 20.4945) -> (48.7105, 22.1254) centre (38.1485, 31.6326) ccw projected
  arc A339 (48.7105, 22.1254) -> (48.3741, 22.8516) centre (0, 0) ccw projected
  arc A340 (48.3741, 22.8516) -> (46.007, 22.5813) centre (48.7971, 8.6472) ccw projected
  arc A341 (46.007, 22.5813) -> (45.6641, 23.267) centre (0, 0) ccw projected
  arc A342 (45.6641, 23.267) -> (47.3002, 24.9989) centre (36.1885, 33.8574) ccw projected
  arc A343 (47.3002, 24.9989) -> (46.9209, 25.7037) centre (0, 0) ccw projected
  arc A344 (46.9209, 25.7037) -> (44.5742, 25.2923) centre (48.1926, 11.55) ccw projected
  arc A345 (44.5742, 25.2923) -> (44.1909, 25.9563) centre (0, 0) ccw projected
  arc A346 (44.1909, 25.9563) -> (45.7205, 27.7829) centre (34.0989, 35.961) ccw projected
  arc A347 (45.7205, 27.7829) -> (45.2997, 28.4637) centre (0, 0) ccw projected
  arc A348 (45.2997, 28.4637) -> (42.9819, 27.9128) centre (47.4156, 14.4114) ccw projected
  arc A349 (42.9819, 27.9128) -> (42.5595, 28.5526) centre (0, 0) ccw projected
  arc A350 (42.5595, 28.5526) -> (43.9771, 30.4674) centre (31.8872, 37.9359) ccw projected
  arc A351 (43.9771, 30.4674) -> (43.5164, 31.1219) centre (0, 0) ccw projected
  arc A352 (43.5164, 31.1219) -> (41.2356, 30.4333) centre (46.4689, 17.2213) ccw projected
  arc A353 (41.2356, 30.4333) -> (40.7758, 31.0467) centre (0, 0) ccw projected
  arc A354 (40.7758, 31.0467) -> (42.0763, 33.0429) centre (29.5614, 39.775) ccw projected
  arc A355 (42.0763, 33.0429) -> (41.5773, 33.6686) centre (0, 0) ccw projected
  arc A356 (41.5773, 33.6686) -> (39.3418, 32.8449) centre (45.3558, 19.9695) ccw projected
  arc A357 (39.3418, 32.8449) -> (38.8461, 33.4297) centre (0, 0) ccw projected
  arc A358 (38.8461, 33.4297) -> (40.0249, 35.5001) centre (27.1298, 41.4717) ccw projected
  arc A359 (40.0249, 35.5001) -> (39.4894, 36.0949) centre (0, 0) ccw projected
  arc A360 (39.4894, 36.0949) -> (37.3071, 35.1389) centre (44.0803, 22.6462) ccw projected
  arc A361 (37.3071, 35.1389) -> (36.7773, 35.6931) centre (0, 0) ccw projected
  arc A362 (36.7773, 35.6931) -> (37.8302, 37.8302) centre (24.6011, 43.0199) ccw projected
  arc A363 (37.8302, 37.8302) -> (37.2601, 38.3919) centre (0, 0) ccw projected
  arc A364 (37.2601, 38.3919) -> (35.1389, 37.3071) centre (42.6471, 25.2419) ccw projected
  arc A365 (35.1389, 37.3071) -> (34.5769, 37.8286) centre (0, 0) ccw projected
  arc A366 (34.5769, 37.8286) -> (35.5001, 40.0249) centre (21.9843, 44.4142) ccw projected
  arc A367 (35.5001, 40.0249) -> (34.8974, 40.5515) centre (0, 0) ccw projected
  arc A368 (34.8974, 40.5515) -> (32.8449, 39.3418) centre (41.0612, 27.7472) ccw projected
  arc A369 (32.8449, 39.3418) -> (32.2527, 39.8287) centre (0, 0) ccw projected
  arc A370 (32.2527, 39.8287) -> (33.0429, 42.0763) centre (19.2888, 45.6494) ccw projected
  arc A371 (33.0429, 42.0763) -> (32.4098, 42.5659) centre (0, 0) ccw projected
  arc A372 (32.4098, 42.5659) -> (30.4333, 41.2356) centre (39.3283, 30.1531) ccw projected
  arc A373 (30.4333, 41.2356) -> (29.813, 41.6863) centre (0, 0) ccw projected
  arc A374 (29.813, 41.6863) -> (30.4674, 43.9771) centre (16.5242, 46.7213) ccw projected
  arc A375 (30.4674, 43.9771) -> (29.8061, 44.428) centre (0, 0) ccw projected
  arc A376 (29.8061, 44.428) -> (27.9128, 42.9819) centre (37.4546, 32.4512) ccw projected
  arc A377 (27.9128, 42.9819) -> (27.2666, 43.3946) centre (0, 0) ccw projected
  arc A378 (27.2666, 43.3946) -> (27.7829, 45.7205) centre (13.7005, 47.6259) ccw projected
  arc A379 (27.7829, 45.7205) -> (27.0958, 46.131) centre (0, 0) ccw projected
  arc A380 (27.0958, 46.131) -> (25.2923, 44.5742) centre (35.4469, 34.633) ccw projected
  arc A381 (25.2923, 44.5742) -> (24.6227, 44.9476) centre (0, 0) ccw projected
  arc A382 (24.6227, 44.9476) -> (24.9989, 47.3002) centre (10.8278, 48.36) ccw projected
  arc A383 (24.9989, 47.3002) -> (24.2885, 47.6688) centre (0, 0) ccw projected
  arc A384 (24.2885, 47.6688) -> (22.5813, 46.007) centre (33.3122, 36.6909) ccw projected
  arc A385 (22.5813, 46.007) -> (21.8905, 46.3397) centre (0, 0) ccw projected
  arc A386 (21.8905, 46.3397) -> (22.1254, 48.7105) centre (7.9163, 48.921) ccw projected
  arc A387 (22.1254, 48.7105) -> (21.3942, 49.0361) centre (0, 0) ccw projected
  arc A388 (21.3942, 49.0361) -> (19.7895, 47.2751) centre (31.0583, 38.6174) ccw projected
  arc A389 (19.7895, 47.2751) -> (19.08, 47.5659) centre (0, 0) ccw projected
  arc A390 (19.08, 47.5659) -> (19.1727, 49.9466) centre (4.9764, 49.3068) ccw projected
  arc A391 (19.1727, 49.9466) -> (18.4234, 50.2278) centre (0, 0) ccw projected
  arc A392 (18.4234, 50.2278) -> (16.9268, 48.374) centre (28.6933, 40.4057) ccw projected
  arc A393 (16.9268, 48.374) -> (16.2013, 48.6218) centre (0, 0) ccw projected
  arc A394 (16.2013, 48.6218) -> (16.1514, 51.0038) centre (2.0188, 49.5162) ccw projected
  arc A395 (16.1514, 51.0038) -> (15.3866, 51.2397) centre (0, 0) ccw projected
  arc A396 (15.3866, 51.2397) -> (14.0035, 49.2997) centre (26.2255, 42.0494) ccw projected
  arc A397 (14.0035, 49.2997) -> (13.2645, 49.5037) centre (0, 0) ccw projected
  arc A398 (13.2645, 49.5037) -> (13.0722, 51.8784) centre (-0.9461, 49.5483) ccw projected
  arc A399 (13.0722, 51.8784) -> (12.2947, 52.0681) centre (0, 0) ccw projected
  arc A400 (12.2947, 52.0681) -> (11.0301, 50.049) centre (23.6638, 43.5425) ccw projected
  arc A401 (11.0301, 50.049) -> (10.2802, 50.2084) centre (0, 0) ccw projected
  arc A402 (10.2802, 50.2084) -> (9.9463, 52.5673) centre (-3.9076, 49.403) ccw projected
  arc A403 (9.9463, 52.5673) -> (9.1588, 52.7102) centre (0, 0) ccw projected
  arc A404 (9.1588, 52.7102) -> (8.0173, 50.619) centre (21.0174, 44.8798) ccw projected
  arc A405 (8.0173, 50.619) -> (7.2591, 50.7333) centre (0, 0) ccw projected
  arc A406 (7.2591, 50.7333) -> (6.7847, 53.068) centre (-6.8551, 49.0809) ccw projected
  arc A407 (6.7847, 53.068) -> (5.9901, 53.1636) centre (0, 0) ccw projected
  arc A408 (5.9901, 53.1636) -> (4.9757, 51.0079) centre (18.2958, 46.0564) ccw projected
  arc A409 (4.9757, 51.0079) -> (4.2121, 51.0766) centre (0, 0) ccw projected
  arc A410 (4.2121, 51.0766) -> (3.5989, 53.3788) centre (-9.7781, 48.5831) ccw projected
  arc A411 (3.5989, 53.3788) -> (2.8, 53.4267) centre (0, 0) ccw projected
  arc A412 (2.8, 53.4267) -> (1.9163, 51.2142) centre (15.5087, 47.0681) ccw projected
  arc A413 (1.9163, 51.2142) -> (1.15, 51.2371) centre (0, 0) ccw projected
  arc A414 (1.15, 51.2371) -> (0.4002, 53.4985) centre (-12.6661, 47.9114) ccw projected
  arc A415 (0.4002, 53.4985) -> (-0.4002, 53.4985) centre (0, 0) ccw projected
  arc A416 (-0.4002, 53.4985) -> (-1.15, 51.2371) centre (12.6661, 47.9114) ccw projected
  arc A417 (-1.15, 51.2371) -> (-1.9163, 51.2142) centre (0, 0) ccw projected
  arc A418 (-1.9163, 51.2142) -> (-2.8, 53.4267) centre (-15.5087, 47.0681) ccw projected
  arc A419 (-2.8, 53.4267) -> (-3.5989, 53.3788) centre (0, 0) ccw projected
  circle A420 centre (0, 0) radius 65
  dimension "d49" = 130
  constraints: 1 centre point, 1 coincident
  measures "d49" diameter of A420
extrude "擠出2" add sketch "草圖4" against normal blind 15 separate body
equation "\"d0\" = da_da"
equation "\"d1\" = da_b"
equation "\"d3\" = da_dw"
equation "\"d16\" = da_aw"
equation "\"d43\" = da_aw"
equation "\"d46\" = da_aw"
equation "\"da_da\" = 107"
equation "\"da_b\" = 15"
equation "\"da_dw\" = 105"
equation "\"da_aw\" = 81"
body "Solid1"
body "Srf1"
